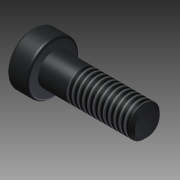
# Autodesk Inventor part: DIN-6912 - M6x18(F)
Saved by Autodesk Inventor 2011 SP1 (Build 150282100, 282)
## iProperties
Created: 2018-05-26
Part Number: DIN-6912 - M6x18(F)
Catalog Web Link: www.cadenas.de
Description: DIN-6912-Hexagon socket head cap screw with centre hole and low head
Vendor: FESTO
Document SubType Name: Modeling
Designer: psAdmin
Manufacturer: FESTO
Mass: 0.734713 g
Surface Area: 6.64112 cm^2
Volume: 0.734713 cm^3
Density: 1 g/cm^3
Category: PARTsolutions
Company: FESTO
Title: DIN-6912 - M6x18(F)
Author: Cadenas PARTsolutions
Comments: Hexagon socket head cap screw with centre hole and low head
PSOL_IDENT_0: {$CADENAS_DATA\23d-libs\festo\zyl_zubeh\din_6912\din_6912.prj},184 {VTYP=3D},{NB=DIN-6912 - M6x18(F)
PSOL_IDENT_1: },{LINA=DIN-6912 - M6x18(F)},{NN=DIN-6912},{DATE=16.11.2017 11:29:57},{GEOMDATE=16.11.2017 11:29:44}
PSOL_IDENT_2: ,{VERSION=},{LINEID=1170},{LINESUBID=-1},{WBVAR=}  {NB=DIN-6912 - M6x18(F)},{LINA=DIN-6912 - M6x18(F
PSOL_IDENT_3: )},{KT=L},{IDNR=},{NENN=M6x18},{D=6.000},{L=18.000},{DK=4.773},{LS=2.500},{LG=5.500},{DK1=10.000},{D
PSOL_IDENT_4: H=3.000},{K=4.000},{R=0.250},{V=0.500},{S=5.000},{T1=2.500},{T2=5.000},{F=0.680},{DA=6.800},{DW=9.20
PSOL_IDENT_5: 0}
NN: DIN-6912
NT: Hexagon socket head cap screw with centre hole and low head
NB: DIN-6912 - M6x18(F)
NBSYN: DIN-6912 - $NENN.(F)
LINA: DIN-6912 - M6x18(F)
ROWDESC: M6x18
D: 6.000
L: 18.000
DK: 4.773
LS: 2.500
LG: 5.500
DK1: 10.000
DH: 3.000
K: 4.000
R: 0.250
V: 0.500
S: 5.000
T1: 2.500
T2: 5.000
F: 0.680
DA: 6.800
DW: 9.200
SUPPLIER: FESTO
ARTICLENO: DIN-6912 - M6x18(F)
BOMINFO: DIN-6912 - M6x18(F)
CREATOR: CADENAS GmbH
Autodesk Inventor part; units mm, degrees
sketch "Sketch_1" plane through (0, 0, 0) normal (0, 0, 1) x (1, 0, 0)
  line L0 (18, 0) -> (2.5, 0)
  line L1 (2.5, 0) -> (1, 1.5)
  line L2 (1, 1.5) -> (-0.5, 1.5)
  line L3 (-0.5, 1.5) -> (-1.5, 2.5)
  line L4 (-1.5, 2.5) -> (-3.6132, 2.5)
  line L5 (-3.6132, 2.5) -> (-4, 2.8868)
  line L6 (-4, 2.8868) -> (-4, 4.5)
  arc A0 (-3.5, 5) -> (-4, 4.5) centre (-3.5, 4.5) ccw
  line L7 (-3.5, 5) -> (-0.5, 5)
  arc A1 (0, 4.5) -> (-0.5, 5) centre (-0.5, 4.5) ccw
  line L8 (0, 4.5) -> (0, 3)
  line L9 (0, 3) -> (17.3865, 3)
  line L10 (17.3865, 3) -> (18, 2.3865)
  line L11 (18, 2.3865) -> (18, 0)
  line L12 (18, 0) -> (2.5, 0)
  constraints: 26 end point, 4 point on circle, 2 centre point
revolve "Revolution1" add sketch "Sketch_1" angle 360 about axis through (18, 0, 0) along (-1, 0, 0)
thread "Thread1" size "M6x1" class "6g" standard "ISO Metric profile" length 11.8865
sketch "Sketch_2" plane through (-4, 0, 0) normal (1, 0, 0) x (0, 0, -1)
  line L0 (-2.5, -1.4434) -> (0, -2.8868)
  line L1 (0, -2.8868) -> (2.5, -1.4434)
  line L2 (2.5, -1.4434) -> (2.5, 1.4434)
  line L3 (2.5, 1.4434) -> (0, 2.8868)
  line L4 (0, 2.8868) -> (-2.5, 1.4434)
  line L5 (-2.5, 1.4434) -> (-2.5, -1.4434)
  constraints: 12 end point
extrude "Extrusion1" cut sketch "Sketch_2" along normal blind 2.5
ref_plane "MONTAGE_XY" through (0, 0, 0) normal (1, 0, 0) x (0, 0, -1)
ref_plane "MONTAGE_YZ" through (0, 0, 0) normal (0, 0, -1) x (0, 1, 0)
ref_plane "MONTAGE_ZX" through (0, 0, 0) normal (0, 1, 0) x (1, 0, 0)
ref_plane "Schrauben_punkt_XY" through (18, 0, 0) normal (-1, 0, 0) x (0, 0, -1)
ref_plane "Schrauben_punkt_YZ" through (18, 0, 0) normal (0, 0, -1) x (0, -1, 0)
ref_plane "Schrauben_punkt_ZX" through (18, 0, 0) normal (0, -1, 0) x (-1, 0, 0)
body "Solid1"
